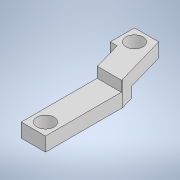
# Autodesk Inventor part: Деталь2
Saved by Autodesk Inventor 2020 (Build 240168000, 168)
## iProperties
Created: 2021-07-20
Part Number: Деталь2
Material: Типовые
Document SubType Name: Modeling
Designer: Антон
Density: 1 g/cm^3
Appearance: По умолчанию
Author: Антон
Autodesk Inventor part; units mm, degrees
ref_plane "YZ Plane" through (0, 0, 0) normal (1, 0, 0) x (0, 1, 0)
ref_plane "XZ Plane" through (0, 0, 0) normal (0, 1, 0) x (-1, 0, 0)
ref_plane "XY Plane" through (0, 0, 0) normal (0, 0, 1) x (1, 0, 0)
sketch "Эскиз1" plane through (0, 0, 0) normal (0, 1, 0) x (-1, 0, 0)
  circle A0 centre (0, 0) radius 2.475
  circle A1 centre (4.15, -29.6507) radius 2.475
  line L0 (0, 0) -> (0, -29.6507) construction
  line L1 (0, -29.6507) -> (4.15, -29.6507) construction
  line L2 (-3.475, -3.475) -> (3.475, -3.475)
  line L3 (3.475, -3.475) -> (3.475, 3.475)
  line L4 (3.475, 3.475) -> (-3.475, 3.475)
  line L5 (-3.475, 3.475) -> (-3.475, -3.475)
  line L6 (-3.475, -3.475) -> (3.475, 3.475) construction
  line L7 (3.475, -3.475) -> (-3.475, 3.475) construction
  line L8 (0.675, -26.1757) -> (7.625, -26.1757)
  line L9 (7.625, -26.1757) -> (7.625, -33.1257)
  line L10 (7.625, -33.1257) -> (0.675, -33.1257)
  line L11 (0.675, -33.1257) -> (0.675, -26.1757)
  line L12 (0.675, -26.1757) -> (7.625, -33.1257) construction
  line L13 (7.625, -26.1757) -> (0.675, -33.1257) construction
  line L14 (0, 3.475) -> (0, 2.475) construction
  line L15 (3.475, -3.475) -> (-3.475, -3.475)
  line L16 (-3.475, -3.475) -> (-3.475, -18.6088)
  line L17 (-3.475, -18.6088) -> (3.475, -18.6088)
  line L18 (3.475, -18.6088) -> (3.475, -3.475)
  line L19 (3.475, -26.1757) -> (3.475, -18.6088)
  line L20 (3.475, -18.6088) -> (3.475, -11.0419)
  line L21 (3.475, -11.0419) -> (3.475, -3.475)
  line L22 (3.475, -18.6088) -> (5.6382, -26.1757)
  line L23 (-3.475, -18.6088) -> (0.675, -33.1257)
  dimension "d0" = 4.95
  dimension "d1" = 4.15
  dimension "d2" = 29.6507
  dimension "d3" = 1
  dimension "d4" = 1
  constraints: 48 end point, 7 parallel, 6 midpoint, 4 equal length, 4 perpendicular, 3 horizontal, 3 vertical, 2 coincident, 2 point on line, 1 centre point, 1 collinear, 1 vertical alignment, 3 other
  measures "d1" distance of L0.end L1.end
  measures "d2" distance of L0.start L0.end
  measures "d3" distance edge to line of A1 L9
  measures "d4" distance of L14.start L14.end
extrude "Выдавливание1" add sketch "Эскиз1" along normal blind 7
sketch "Эскиз2" plane through (3.475, 0, 3.475) normal (1, 0, 0) x (0, 0, -1)
  line L0 (22.0838, 7) -> (0, 7) projected
  line L1 (22.0838, 0) -> (0, 0) projected
  line L2 (0, 0) -> (21.7338, 0)
  line L3 (21.7338, 0) -> (21.7338, 4)
  line L4 (21.7338, 4) -> (0, 4)
  line L5 (0, 4) -> (0, 0)
  line L6 (36.6007, 0) -> (36.6007, 7) projected
  line L7 (36.6007, 7) -> (25.7338, 7)
  line L8 (25.7338, 7) -> (25.7338, 3)
  line L9 (25.7338, 3) -> (36.6007, 3)
  line L10 (36.6007, 3) -> (36.6007, 7)
  line L11 (25.7338, 7) -> (21.7338, 7)
  line L12 (21.7338, 7) -> (21.7338, 0)
  line L13 (21.7338, 0) -> (25.7338, 0)
  line L14 (25.7338, 0) -> (25.7338, 7)
  line L15 (0, 0) -> (22.0838, 0) projected
  line L16 (22.0838, 0) -> (22.0838, 7) projected
  line L17 (0, 7) -> (22.0838, 7) projected
  line L18 (0, 0) -> (0, 7) projected
  line L19 (22.0838, 0) -> (36.6007, 0) projected
  line L20 (36.6007, 0) -> (36.6007, 7) projected
  line L21 (22.0838, 7) -> (36.6007, 7) projected
  line L22 (22.0838, 0) -> (22.0838, 7) projected
  line L23 (0, 0) -> (10.8669, 0)
  line L24 (10.8669, 0) -> (21.7338, 0)
  point P0 (3.475, 0)
  point P1 (29.6507, 7)
  point P2 (29.6507, 0)
  point P3 (0, 4)
  dimension "d8" = 4
  constraints: 28 end point, 11 equal length, 3 horizontal, 3 perpendicular, 1 point on line
  measures "d8" distance of L3.end L2.end
extrude "Выдавливание2" cut sketch "Эскиз2" against normal through all contours L12 L4 L18 L0 | L9 L6 L19 L14
